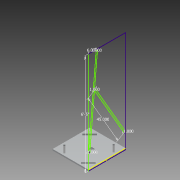
# Autodesk Inventor part: BotLayoutGLass
Saved by Autodesk Inventor 2013 SP2 (Build 170200200, 200)
## iProperties
Created: 2015-01-07
Part Number: BotLayoutGLass
Material: Glass
Document SubType Name: Modeling
Designer: darkb_000
Density: 2.18 g/cm^3
Author: darkb_000
Autodesk Inventor part; units mm, degrees
ref_plane "YZ Plane" through (0, 0, 0) normal (1, 0, 0) x (0, 1, 0)
ref_plane "XZ Plane" through (0, 0, 0) normal (0, 1, 0) x (-1, 0, 0)
ref_plane "XY Plane" through (0, 0, 0) normal (0, 0, 1) x (1, 0, 0)
sketch "Sketch1" plane through (0, 0, 0) normal (0, 1, 0) x (-1, 0, 0)
  line L0 (-342.9, 342.9) -> (342.9, 342.9)
  line L1 (342.9, 342.9) -> (342.9, -342.9)
  line L2 (342.9, -342.9) -> (-342.9, -342.9)
  line L3 (-342.9, -342.9) -> (-342.9, 342.9)
  point P0 (0, 0)
  point P1 (0, 0)
  dimension "d0" = 685.8
  dimension "d1" = 685.8
  constraints: 8 end point, 2 parallel, 1 coincident, 1 horizontal, 1 perpendicular
  measures "d0" distance of L1.end L2.end
  measures "d1" distance of L0.end L1.end
extrude "Extrusion1" add sketch "Sketch1" along normal blind 25.4
sketch "Sketch2" plane through (0, 25.4, 0) normal (0, 1, 0) x (1, 0, 0)
  line L0 (-342.9, -314.325) -> (342.9, -314.325) projected
  line L1 (342.9, 346.075) -> (-342.9, 346.075) projected
  line L2 (-317.5, 346.075) -> (-317.5, -314.325) projected
  line L3 (317.5, -314.325) -> (317.5, 346.075) projected
  line L4 (-342.9, 374.65) -> (342.9, 374.65) projected
  line L5 (-342.9, 342.9) -> (342.9, 342.9)
  line L6 (342.9, 342.9) -> (342.9, 374.65)
  line L7 (342.9, 374.65) -> (-342.9, 374.65)
  line L8 (-342.9, 374.65) -> (-342.9, 342.9)
  point P0 (0, 0)
  constraints: 8 end point, 2 parallel, 1 horizontal, 1 perpendicular
extrude "Extrusion2" add sketch "Sketch2" against normal blind 25.4 contours L5 L8 L1 L2 | L2 L1 L3 L5 | L3 L1 L6 L5 | L1 L8 L4 L6
sketch "Sketch3" plane through (0, 25.4, 0) normal (0, 1, 0) x (1, 0, 0)
  line L0 (342.9, 346.075) -> (-342.9, 346.075) projected
  line L1 (-317.5, 346.075) -> (-317.5, -314.325) projected
  line L2 (317.5, -314.325) -> (317.5, 346.075) projected
  line L3 (-342.9, -314.325) -> (342.9, -314.325) projected
  line L4 (-317.5, 346.075) -> (-76.2, 346.075) construction
  line L5 (-317.5, 346.075) -> (-146.8751, 346.075)
  line L6 (-317.5, 175.4501) -> (-317.5, 346.075)
  line L7 (-151.3653, 323.6244) -> (-169.3258, 341.5849)
  line L8 (-169.3258, 341.5849) -> (-313.0099, 197.9008)
  line L9 (-313.0099, 197.9008) -> (-295.0494, 179.9403)
  line L10 (-295.0494, 179.9403) -> (-151.3653, 323.6244)
  line L11 (151.3653, 323.6244) -> (169.3258, 341.5849)
  line L12 (169.3258, 341.5849) -> (313.0099, 197.9008)
  line L13 (313.0099, 197.9008) -> (295.0494, 179.9403)
  line L14 (295.0494, 179.9403) -> (151.3653, 323.6244)
  line L15 (-151.3653, -291.8744) -> (-169.3258, -309.8349)
  line L16 (-169.3258, -309.8349) -> (-313.0099, -166.1508)
  line L17 (-313.0099, -166.1508) -> (-295.0494, -148.1903)
  line L18 (-295.0494, -148.1903) -> (-151.3653, -291.8744)
  line L19 (295.0494, -148.1903) -> (151.3653, -291.8744)
  line L20 (313.0099, -166.1508) -> (295.0494, -148.1903)
  line L21 (169.3258, -309.8349) -> (313.0099, -166.1508)
  line L22 (151.3653, -291.8744) -> (169.3258, -309.8349)
  point P0 (0, 0)
  dimension "d10" = 25.4
  dimension "d11" = 203.2
  dimension "d12" = 25.4
  constraints: 38 end point, 2 horizontal
  measures "d10" distance of L7.start L7.end
  measures "d11" distance of L7.end L8.end
  measures "d12" distance of L8.end L9.end
extrude "Extrusion3" cut sketch "Sketch3" against normal blind 25.4 contours L10 L9 L8 L7 | L11 L12 L13 L14 | L15 L16 L17 L18 | L20 L21 L22 L19
sketch "Sketch4" plane through (0, 25.4, 0) normal (0, 1, 0) x (1, 0, 0)
  line L0 (342.9, -342.9) -> (342.9, 374.65) projected
  line L1 (-342.9, 374.65) -> (-342.9, -342.9) projected
  line L2 (342.9, 346.075) -> (-342.9, 346.075) projected
  line L3 (-342.9, -314.325) -> (342.9, -314.325) projected
  line L4 (0, 346.075) -> (0, -314.325)
  line L5 (-342.9, 15.875) -> (342.9, 15.875)
  line L6 (0, 15.875) -> (50.8, 15.875)
  line L7 (50.8, 15.875) -> (50.8, 66.675)
  line L8 (50.8, 66.675) -> (0, 66.675)
  line L9 (0, 66.675) -> (0, 15.875)
  point P0 (0, 0)
  dimension "d15" = 50.8
  dimension "d16" = 50.8
  constraints: 12 end point, 5 midpoint, 2 parallel, 1 horizontal, 1 perpendicular
  measures "d15" distance of L8.end L7.end
  measures "d16" distance of L7.end L6.end
extrude "Extrusion4" cut sketch "Sketch4" against normal blind 25.4 contours L5 L4 L8 L7
sketch "Sketch5" plane through (342.9, 0, 342.9) normal (1, 0, 0) x (0, 0, -1)
  line L0 (717.55, 0) -> (0, 0) projected
  line L1 (717.55, 25.4) -> (717.55, 0) projected
  line L2 (0, 25.4) -> (717.55, 25.4) projected
  line L3 (0, 0) -> (0, 25.4) projected
  line L4 (717.55, 0) -> (0, 0)
  line L5 (0, 0) -> (0, 1955.8)
  line L6 (0, 1955.8) -> (717.55, 1955.8)
  line L7 (717.55, 1955.8) -> (717.55, 0)
  line L8 (0, 1955.8) -> (152.4, 1955.8)
  circle A0 centre (15.875, 301.625) radius 3.175 projected
  circle A1 centre (15.875, 301.625) radius 12.7
  line L9 (152.4, 1955.8) -> (3.2264, 302.7664)
  line L10 (152.4, 1955.8) -> (177.6972, 1953.5171)
  line L11 (177.6972, 1953.5171) -> (28.5236, 300.4836)
  circle A2 centre (701.675, 301.625) radius 3.175 projected
  circle A3 centre (701.675, 301.625) radius 12.7
  line L12 (701.675, 301.625) -> (714.375, 301.625) construction
  line L13 (712.6735, 307.975) -> (141.1735, 1297.842)
  line L14 (141.1735, 1297.842) -> (119.1765, 1285.142)
  line L15 (119.1765, 1285.142) -> (690.6765, 295.275)
  point P0 (342.9, 0)
  dimension "d19" = 1955.8
  dimension "d20" = 152.4
  dimension "d21" = 25.4
  dimension "d22" = 25.4
  dimension "d23" = 25.4
  dimension "d25" = 1143
  dimension "d26" = 25.4
  constraints: 24 end point, 4 point on circle, 4 tangent, 3 perpendicular, 2 centre point, 2 coincident, 2 horizontal, 2 parallel, 1 point on line
  measures "d19" distance of L4.end L5.end
  measures "d20" distance of L5.end L8.end
  measures "d21" diameter of A1
  measures "d22" distance of L8.end L10.end
  measures "d23" diameter of A3
  measures "d25" distance of L13.start L13.end
  measures "d26" distance of L13.end L14.end
body "Solid1"
